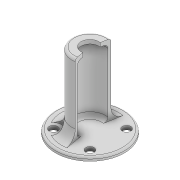
# Autodesk Inventor part: Tool1
Saved by Autodesk Inventor 2021 (Build 250183000, 183)
## iProperties
Created: 2022-10-21
Part Number: Tool1
Material: Generic
Document SubType Name: Modeling
Designer: brian
Density: 1 g/cm^3
Appearance: Default
Mass: 12.4385 g
Surface Area: 101.981 cm^2
Volume: 12.4385 cm^3
Author: brian
## iProperties of the stored document _3DPrint.ipt
Created: 2022-11-02
Part Number: _3DPrint
Material: Generic
Document SubType Name: Modeling
Designer: brian
Density: 1 g/cm^3
Appearance: Default
Author: brian
Autodesk Inventor part; units mm, degrees
ref_plane "YZ Plane" through (0, 0, 0) normal (1, 0, 0) x (0, 1, 0)
ref_plane "XZ Plane" through (0, 0, 0) normal (0, 1, 0) x (-1, 0, 0)
ref_plane "XY Plane" through (0, 0, 0) normal (0, 0, 1) x (1, 0, 0)
sketch "Sketch1" plane through (0, 0, 0) normal (0, 1, 0) x (-1, 0, 0)
  circle A0 centre (0, 0) radius 26.5
  circle A1 centre (-14.1421, 14.1421) radius 3.25
  circle A2 centre (-14.1421, -14.1421) radius 3.25
  circle A3 centre (14.1421, -14.1421) radius 3.25
  circle A4 centre (14.1421, 14.1421) radius 3.25
  line L0 (0, 0) -> (0, 26.5) construction
  line L1 (0, 0) -> (-18.7383, 18.7383) construction
  dimension "d0" = 53
  dimension "d1" = 6.5
  dimension "d2" = 20
  dimension "d5" = 360
  dimension "d9" = 45
  constraints: 5 centre point, 4 end point, 2 point on circle, 1 coincident, 1 point on line, 1 vertical, 9 other
  measures "d0" diameter of A0
  measures "d1" diameter of A1
  measures "d2" distance of A1.centre point (0, 0)
  measures "d9" angle of L1 L0
extrude "Extrusion1" add sketch "Sketch1" along normal blind 3
sketch "Sketch2" plane through (0, 0, 0) normal (0, 0, 1) x (1, 0, 0)
  line L0 (26.5, 3) -> (-26.5, 3) projected
  line L1 (-12, 3) -> (-14, 3)
  line L2 (-14, 3) -> (-14, 58)
  line L3 (-14, 58) -> (-12, 58)
  line L4 (-12, 58) -> (-12, 3)
  line L5 (-14, 58) -> (-6.85, 58)
  line L6 (-6.85, 58) -> (-6.85, 55)
  line L7 (-6.85, 55) -> (-14, 55)
  line L8 (-14, 55) -> (-14, 58)
  line L9 (0, -11.6) -> (0, 69.6) projected
  point P0 (0, 0)
  point P1 (-12, 55)
  dimension "d10" = 12
  dimension "d11" = 6.85
  dimension "d12" = 2
  dimension "d13" = 55
  dimension "d14" = 3
  constraints: 16 end point, 4 parallel, 2 horizontal, 2 perpendicular, 1 point on line
  measures "d10" horizontal distance of point (0, 0) L1.start
  measures "d11" horizontal distance of point (0, 0) L5.end
  measures "d12" distance between parallel lines of L2 L4
  measures "d13" distance between parallel lines of L0 L5
  measures "d14" distance of L5.end L6.end
revolve "Revolution1" add sketch "Sketch2" angle 200 mid plane about axis through (0, -10, 0) along (0, 1, 0)
fillet "Fillet1" radius 8 1 edges at (-14, 3, 0)
fillet "Fillet1" radius 3 1 edges at (-12, 55, 0)
fillet "Fillet1" radius 3 1 edges at (-12, 3, 0)
fillet "Fillet1" radius 2 1 edges at (-14, 58, 0)
fillet "Fillet1" radius 1.5 1 edges at (26.5, 3, 0)
sketch "Sketch3" plane through (0, 3, 0) normal (0, 1, 0) x (1, 0, 0)
  circle A0 centre (14.1421, 14.1421) radius 3.25 projected
  circle A1 centre (14.1421, 14.1421) radius 6
  circle A2 centre (-14.1421, 14.1421) radius 6
  circle A3 centre (-14.1421, -14.1421) radius 6
  circle A4 centre (14.1421, -14.1421) radius 6
  arc A5 (2.4311, 13.7873) -> (2.4311, -13.7873) centre (0, 0) ccw projected
  dimension "d23" = 360
  dimension "d27" = 12
  constraints: 4 centre point, 1 coincident, 9 other
  measures "d27" diameter of A1
extrude "Extrusion2" cut sketch "Sketch3" along normal blind 8 contours A0 | A1 | A2 | A3 | A4
body "Solid1"
